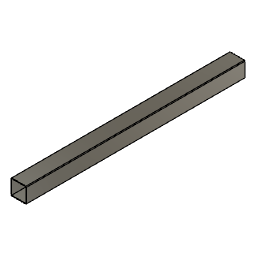
_Profil50x50_700mm.639981a4-a0fb-4878-b3d5-07ecfbe12696 (Autodesk Fusion 360 design; units mm, degrees)
Autodesk Fusion 360 part; units mm, degrees
note: some values were not read from the file. Set by a fixed rule: which sketch regions a step uses.
sketch "Sketch1" plane through (0, 0, 0) normal (0, 1, 0) x (1, 0, 0)
  line L0 (0, -25) -> (23, -25)
  line L1 (25, -23) -> (25, 23)
  line L2 (23, 25) -> (0, 25)
  line L3 (0, -25) -> (-23, -25)
  line L4 (-25, -23) -> (-25, 23)
  line L5 (-23, 25) -> (0, 25)
  line L6 (0, -23) -> (-23, -23)
  line L7 (-23, -23) -> (-23, 23)
  line L8 (-23, 23) -> (0, 23)
  line L9 (23, 23) -> (0, 23)
  line L10 (23, -23) -> (23, 23)
  line L11 (0, -23) -> (23, -23)
  arc A0 (23, -25) -> (25, -23) centre (23, -23) ccw
  arc A1 (-25, -23) -> (-23, -25) centre (-23, -23) ccw
  arc A2 (-23, 25) -> (-25, 23) centre (-23, 23) ccw
  arc A3 (25, 23) -> (23, 25) centre (23, 23) ccw
  point P0 (25, -25)
  point P1 (25, 25)
  dimension "d1" = 25
  dimension "d2" = 25
  dimension "d3" = 50
  dimension "d4" = 2
  dimension "d7" = 2
  dimension "d8" = 2
  dimension "d9" = 2
  dimension "d10" = 2
  constraint horizontal L0
  constraint vertical L1
  constraint horizontal L2
  constraint coincident P0 L0
  constraint coincident P0 L1
  constraint tangent L0 A0
  constraint tangent L1 A0
  constraint tangent L3 A1
  constraint tangent L4 A1
  constraint tangent L4 A2
  constraint tangent L5 A2
  constraint coincident P1 L1
  constraint coincident P1 L2
  constraint tangent L1 A3
  constraint tangent L2 A3
  measures "d1" distance of origin L0.start
  measures "d2" distance of L0.start P0
  measures "d3" distance of P0 P1
  measures "d7" radius of A0
  measures "d8" radius of A1
  measures "d9" radius of A2
  measures "d10" radius of A3
extrude "Extrude1" add sketch "Sketch1" along normal blind 700
